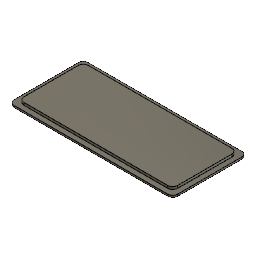
CoverForElectronicsCompartmentBase (Autodesk Fusion 360 design; units mm, degrees)
Autodesk Fusion 360 part; units mm, degrees
sketch "Sketch1" plane through (0, 0, 0) normal (0, 1, 0) x (1, 0, 0)
  line L0 (76.5, -32) -> (-76.5, -32)
  line L1 (-76.5, -32) -> (-76.5, 32)
  line L2 (-76.5, 32) -> (76.5, 32)
  line L3 (76.5, 32) -> (76.5, -32)
  line L4 (76.5, -32) -> (-76.5, 32) construction
  line L5 (-76.5, -32) -> (76.5, 32) construction
  line L6 (81.5, -37) -> (-81.5, -37)
  line L7 (-81.5, -37) -> (-81.5, 37)
  line L8 (-81.5, 37) -> (81.5, 37)
  line L9 (81.5, 37) -> (81.5, -37)
  circle A0 centre (-71.5, 27) radius 5
  circle A1 centre (71.5, 27) radius 5
  circle A2 centre (71.5, -27) radius 5
  circle A3 centre (-71.5, -27) radius 5
  dimension "d1" = 153
  dimension "d2" = 64
  dimension "d4" = -5
  constraint perpendicular L0 L1
  constraint parallel L0 L2
  constraint parallel L1 L3
  constraint horizontal L0
  constraint coincident L4 origin
  constraint coincident L5 origin
  constraint tangent L1 A0
  constraint tangent L3 A1
  constraint tangent L0 A2
  constraint tangent L0 A3
  measures "d1" distance of L1.end L2.end
  measures "d2" distance of L0.end L1.end
extrude "Extrude1" add sketch "Sketch1" along normal blind 2.5 contours L0 L1 L2 L3 A0 A1 A2 A3 | A2 | A3 | A1 | A0
extrude "Extrude2" add sketch "Sketch1" 1 faces at (23.8333, 0, 10.6667) against normal blind 2 contours L0 L3 A2 | L0 L1 L2 L3 A0 A1 A2 A3 | A2 | L0 L1 A3 | A3 | L2 L3 A1 | A1 | L1 L2 A0 | A0 | L6 L7 L8 L9
fillet "Fillet1" radius 5 4 edges at (81.5, -1, 37) (-81.5, -1, 37) (81.5, -1, -37) (-81.5, -1, -37)
